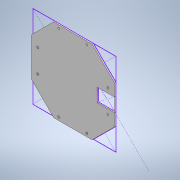
# Autodesk Inventor part: t960_power_distribution_board_TL2996_bottom
Saved by Autodesk Inventor 2020.2 (Build 242310000, 310)
## iProperties
Created: 2020-08-20
Part Number: t960_power_distribution_board_TL2996_bottom
Material: Generic
Document SubType Name: Modeling
Designer: Krishna Makhija
Density: 1 g/cm^3
Appearance: Default
Author: Krishna Makhija
Autodesk Inventor part; units mm, degrees
ref_plane "YZ Plane" through (0, 0, 0) normal (1, 0, 0) x (0, 1, 0)
ref_plane "XZ Plane" through (0, 0, 0) normal (0, 1, 0) x (-1, 0, 0)
ref_plane "XY Plane" through (0, 0, 0) normal (0, 0, 1) x (1, 0, 0)
sketch "Sketch1" plane through (0, 0, 0) normal (0, 0, 1) x (1, 0, 0)
  line L0 (-65.00021, 64.999866) -> (65.00021, 64.999866)
  line L1 (65.00021, 64.999866) -> (65.00021, -64.999866)
  line L2 (65.00021, -64.999866) -> (-65.00021, -64.999866)
  line L3 (-65.00021, -64.999866) -> (-65.00021, 64.999866)
  line L4 (-65.00021, 64.999866) -> (65.00021, -64.999866) construction
  line L5 (65.00021, 64.999866) -> (-65.00021, -64.999866) construction
  line L6 (29.999974, -64.999866) -> (65.00021, -29.999445)
  line L7 (-29.999622, -64.999866) -> (-65.00021, -29.999464)
  line L8 (-29.999622, 64.999866) -> (-65.00021, 29.999464)
  line L9 (29.998617, 64.999866) -> (65.00021, 29.998087)
  line L10 (-13.50021, 64.999866) -> (116.50021, -64.999866) construction
  line L11 (64.999934, -10.4998) -> (38.000066, -10.4998)
  line L12 (38.000066, -10.4998) -> (38.000066, 10.4998)
  line L13 (38.000066, 10.4998) -> (64.999934, 10.4998)
  line L14 (64.999934, 10.4998) -> (64.999934, -10.4998)
  line L15 (64.999934, -10.4998) -> (38.000066, 10.4998) construction
  line L16 (38.000066, -10.4998) -> (64.999934, 10.4998) construction
  line L17 (-38.000066, -10.4998) -> (-64.999934, -10.4998)
  line L18 (-64.999934, -10.4998) -> (-64.999934, 10.4998)
  line L19 (-64.999934, 10.4998) -> (-38.000066, 10.4998)
  line L20 (-38.000066, 10.4998) -> (-38.000066, -10.4998)
  line L21 (-38.000066, -10.4998) -> (-64.999934, 10.4998) construction
  line L22 (-64.999934, -10.4998) -> (-38.000066, 10.4998) construction
  line L23 (16.970375, 2.121415) -> (-2.121415, -16.970375)
  line L24 (-2.121415, -16.970375) -> (-16.970375, -2.121415)
  line L25 (-16.970375, -2.121415) -> (2.121415, 16.970375)
  line L26 (2.121415, 16.970375) -> (16.970375, 2.121415)
  line L27 (-2.121415, -16.970375) -> (2.121415, 16.970375) construction
  constraints: 56 end point, 8 parallel, 8 point on line, 7 perpendicular, 3 horizontal
extrude "Extrusion1" add sketch "Sketch1" along normal blind 2 contours L0 L9 L1 L13 L12 L11 L6 L2 L7 L3 L17 L20 L19 L8 | L19 L20 L17 L3 | L1 L11 L12 L13 | L23 L24 L25 L26
sketch "Sketch2" plane through (0, 0, 2) normal (0, 0, 1) x (1, 0, 0)
  circle A0 centre (22, 60) radius 1.499868
  circle A1 centre (-22, 60) radius 1.499868
  circle A2 centre (22, -60) radius 1.499868
  circle A3 centre (-22, -60) radius 1.499868
  circle A4 centre (55, 18) radius 1.499868
  circle A5 centre (55, -18) radius 1.499868
  circle A6 centre (-55, 18) radius 1.499868
  circle A7 centre (-54.942641, 18) radius 1.499868
  circle A8 centre (-55, -18) radius 1.499868
  circle A9 centre (-54.942641, -18) radius 1.499868
  point P0 (-54.971321, 16.500406)
  point P1 (-54.971321, 19.499594)
  point P2 (-54.971321, -19.499594)
  point P3 (-54.971321, -16.500406)
  constraints: 10 centre point
extrude "Extrusion2" cut sketch "Sketch2" against normal blind 10
sketch "Sketch1 outline for Extrusion3" plane through (0, 0, 0) normal (0, 0, 1) x (1, 0, 0)
  line L0 (64.999934, -10.4998) -> (64.999934, 10.4998)
  line L1 (38.000066, -10.4998) -> (64.999934, -10.4998)
  line L2 (38.000066, 10.4998) -> (38.000066, -10.4998)
  line L3 (64.999934, 10.4998) -> (38.000066, 10.4998)
extrude "Extrusion3" cut sketch "Sketch1 outline for Extrusion3" along normal blind 10
body "Solid1"
